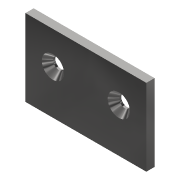
# Autodesk Inventor part: Jaw_Plate
Saved by Autodesk Inventor 2022 (Build 260148000, 148)
## iProperties
Created: 2006-01-18
Part Number: Jaw_Plate
Document SubType Name: Modeling
Designer: PMiller
Material: Steel, High Strength Low Alloy
Density: 7.84 g/cm^3
Appearance: Steel - Polished
Author: PMiller
Autodesk Inventor part; units mm, degrees
ref_plane "YZ Plane" through (0, 0, 0) normal (1, 0, 0) x (0, 1, 0)
ref_plane "XZ Plane" through (0, 0, 0) normal (0, 1, 0) x (-1, 0, 0)
ref_plane "XY Plane" through (0, 0, 0) normal (0, 0, 1) x (1, 0, 0)
sketch "Sketch1" plane through (0, 0, 0) normal (0, 0, 1) x (1, 0, 0)
  line L0 (-34.925, 22.225) -> (34.925, 22.225)
  line L1 (34.925, 22.225) -> (34.925, -22.225)
  line L2 (34.925, -22.225) -> (-34.925, -22.225)
  line L3 (-34.925, -22.225) -> (-34.925, 22.225)
  point P0 (0, 0)
  dimension "d0" = 69.85
  dimension "d1" = 44.45
  dimension "d2" = 34.925
  dimension "d3" = 22.225
  constraints: 8 end point, 2 parallel, 1 horizontal, 1 perpendicular
  measures "d0" distance between parallel lines of L1 L3
  measures "d1" distance between parallel lines of L0 L2
  measures "d2" distance from line of point (0, 0) L1
  measures "d3" distance from line of point (0, 0) L0
extrude "Extrusion1" add sketch "Sketch1" along normal mid plane 4.7625
sketch "Sketch2" plane through (0, 0, 2.3813) normal (0, 0, 1) x (1, 0, 0)
  line L0 (-34.925, -22.225) -> (-34.925, 22.225) projected
  line L1 (34.925, -22.225) -> (-34.925, -22.225) projected
  point P0 (-19.05, 3.175)
  point P1 (19.05, 3.175)
  dimension "d6" = 25.4
  dimension "d7" = 15.875
  dimension "d8" = 38.1
  constraints: 1 horizontal alignment
  measures "d6" distance from line of L1 point (-19.05, 3.175)
  measures "d7" distance from line of L0 point (-19.05, 3.175)
  measures "d8" distance of point (19.05, 3.175) point (-19.05, 3.175)
hole "Hole1" at (-19.05, 3.175, 2.3813) at (19.05, 3.175, 2.3813) direction (0, 0, -1) diameter 6.7564 depth 19.05 tip angle 118 countersink diameter 12.8778 countersink angle 82 clearance for "Flat Head Machine Screw (82)" size "1/4" standard "Ansi Unified Screw Threads"
equation "\"d2\" = 0.5 * d0"
equation "\"d3\" = 0.5 * d1"
body "Solid1"
